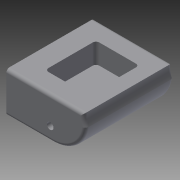
# Autodesk Inventor part: Body
Saved by Autodesk Inventor 2015 (Build 190159000, 159)
## iProperties
Created: 2014-10-28
Part Number: Body
Material: Generic
Document SubType Name: Modeling
Designer: bminden882
Density: 1 g/cm^3
Appearance: Default
Author: bminden882
Autodesk Inventor part; units mm, degrees
ref_plane "YZ Plane" through (0, 0, 0) normal (1, 0, 0) x (0, 1, 0)
ref_plane "XZ Plane" through (0, 0, 0) normal (0, 1, 0) x (-1, 0, 0)
ref_plane "XY Plane" through (0, 0, 0) normal (0, 0, 1) x (1, 0, 0)
sketch "Sketch1" plane through (0, 0, 0) normal (0, 0, 1) x (1, 0, 0)
  line L0 (0, 0) -> (0, 38.608)
  line L1 (0, 38.608) -> (73.787, 38.608)
  arc A0 (73.787, 38.608) -> (75.3246, 27.2) centre (97.4163, 35.9853) ccw
  line L2 (0, 0) -> (44.45, 0)
  arc A1 (44.45, 0) -> (75.3246, 27.2) centre (44.45, 31.1228) ccw
  dimension "d1" = 38.608
  dimension "d2" = 73.787
  dimension "d7" = 44.45
  constraints: 6 end point, 5 point on circle, 2 centre point, 1 horizontal, 1 perpendicular, 1 tangent, 1 vertical
  measures "d1" distance of L0.start L0.end
  measures "d2" distance of L0.end L1.end
  measures "d7" distance of L0.start L2.end
extrude "Extrusion1" add sketch "Sketch1" along normal blind 83.693
sketch "Sketch2" plane through (0, 38.608, 0) normal (0, 1, 0) x (1, 0, 0)
  line L0 (0, 0) -> (0, -83.693) projected
  line L1 (0, 0) -> (73.787, 0) projected
  line L2 (0, 0) -> (0, -83.693) projected
  line L3 (73.787, -83.693) -> (0, -83.693) projected
  line L4 (73.787, 0) -> (73.787, -83.693) projected
  line L5 (73.787, 0) -> (73.787, -83.693) projected
  line L6 (73.787, -17.653) -> (60.198, -17.653)
  line L7 (22.352, -17.653) -> (57.023, -17.653)
  line L8 (60.198, -20.828) -> (60.198, -62.865)
  line L9 (57.023, -66.04) -> (22.352, -66.04)
  line L10 (19.177, -62.865) -> (19.177, -20.828)
  arc A0 (22.352, -17.653) -> (19.177, -20.828) centre (22.352, -20.828) ccw
  arc A1 (60.198, -20.828) -> (57.023, -17.653) centre (57.023, -20.828) ccw
  arc A2 (19.177, -62.865) -> (22.352, -66.04) centre (22.352, -62.865) ccw
  arc A3 (57.023, -66.04) -> (60.198, -62.865) centre (57.023, -62.865) ccw
  point P0 (19.177, -17.653)
  point P1 (60.198, -66.04)
  point P2 (19.177, -66.04)
  dimension "d13" = 13.589
  dimension "d14" = 48.387
  dimension "d26" = 41.021
  dimension "d29" = 3.175
  constraints: 10 end point, 9 point on line, 8 point on circle, 8 tangent, 4 centre point, 3 equal radius, 2 parallel, 1 horizontal, 1 perpendicular
  measures "d13" distance of L6.start L6.end
  measures "d14" distance of point (60.198, -17.653) point (60.198, -66.04)
  measures "d26" distance of point (19.177, -17.653) point (60.198, -17.653)
  measures "d29" radius of A0
extrude "Extrusion2" cut sketch "Sketch2" against normal blind 19.05 contours L7 A1 L8 A3 L9 A2 L10 A0
sketch "Sketch3" plane through (0, 0, 0) normal (-1, 0, 0) x (0, 0, 1)
  line L0 (0, 0) -> (0, 38.608) projected
  line L1 (0, 0) -> (83.693, 0) projected
  line L2 (83.693, 38.608) -> (83.693, 0) projected
  line L3 (0, 38.608) -> (83.693, 38.608) projected
  line L4 (0, 38.608) -> (83.693, 38.608) projected
  line L5 (8.9535, 10.1981) -> (8.9535, 28.3591)
  line L6 (12.1285, 7.0231) -> (71.6915, 7.0231)
  line L7 (74.8665, 10.1981) -> (74.8665, 28.3591)
  line L8 (71.6915, 31.5341) -> (12.1285, 31.5341)
  arc A0 (74.8665, 28.3591) -> (71.6915, 31.5341) centre (71.6915, 28.3591) ccw
  arc A1 (12.1285, 31.5341) -> (8.9535, 28.3591) centre (12.1285, 28.3591) ccw
  arc A2 (8.9535, 10.1981) -> (12.1285, 7.0231) centre (12.1285, 10.1981) ccw
  arc A3 (71.6915, 7.0231) -> (74.8665, 10.1981) centre (71.6915, 10.1981) ccw
  point P0 (8.9535, 7.0231)
  point P1 (8.9535, 31.5341)
  point P2 (74.8665, 7.0231)
  point P3 (74.8665, 31.5341)
  dimension "d20" = 24.511
  dimension "d21" = 65.913
  dimension "d28" = 3.175
  constraints: 8 end point, 8 point on circle, 8 point on line, 8 tangent, 4 centre point, 3 equal radius, 2 perpendicular, 1 horizontal
  measures "d20" distance of point (8.953, 7.023) point (8.953, 31.534)
  measures "d21" distance of point (8.953, 7.023) point (74.866, 7.023)
  measures "d28" radius of A0
extrude "Extrusion3" cut sketch "Sketch3" against normal blind 19.05 contours L5 A1 L8 A0 L7 A3 L6 A2
fillet "Fillet2" radius 3.175 8 edges at (36.8935, 38.608, 83.693) (36.8935, 38.608, 0) (73.8549, 32.8095, 83.693) (22.225, 0, 83.693) (65.0236, 7.7699, 83.693) (73.8549, 32.8095, 0) (22.225, 0, 0) (65.0236, 7.7699, 0)
sketch "Sketch4" plane through (0, 0, 83.693) normal (0, 0, 1) x (1, 0, 0)
  circle A0 centre (41.6613, 12.7) radius 3.175
  line L0 (0, 0) -> (44.45, 0) projected
  dimension "d31" = 6.35
  dimension "d32" = 12.7
  constraints: 1 centre point
  measures "d31" diameter of A0
  measures "d32" distance from line of L0 A0.centre
extrude "Extrusion4" cut sketch "Sketch4" against normal through all
body "Solid1"
